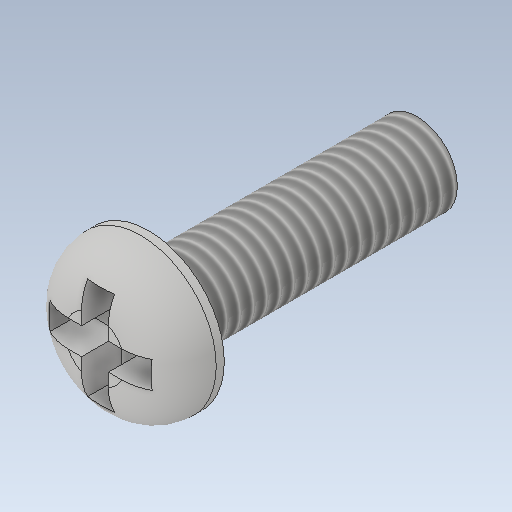
# Autodesk Inventor part: Винт М3х10
Saved by Autodesk Inventor 2020 (Build 240168000, 168)
## iProperties
Created: 2020-03-03
Part Number: Винт М3х10
Material: Типовые
Document SubType Name: Modeling
Designer: Leancher
Density: 1 g/cm^3
Appearance: По умолчанию
Author: Leancher
Autodesk Inventor part; units mm, degrees
ref_plane "YZ Plane" through (0, 0, 0) normal (1, 0, 0) x (0, 1, 0)
ref_plane "XZ Plane" through (0, 0, 0) normal (0, 1, 0) x (-1, 0, 0)
ref_plane "XY Plane" through (0, 0, 0) normal (0, 0, 1) x (1, 0, 0)
sketch "Эскиз1" plane through (0, 0, 0) normal (0, 0, 1) x (1, 0, 0)
  circle A0 centre (-4.8391, -17.7214) radius 1.5
  point P0 (0, 0)
  constraints: 1 centre point
extrude "Выдавливание1" add sketch "Эскиз1" against normal blind 10
sketch "Эскиз2" plane through (-4.8391, -17.7214, 0) normal (0, 0, 1) x (1, 0, 0)
  circle A0 centre (0, 0) radius 2.816
  point P0 (4.8391, 17.7214)
  constraints: 1 centre point
extrude "Выдавливание2" add sketch "Эскиз2" along normal blind 2
fillet "Сопряжение1" radius 1.7 1 edges at (-7.6551, -17.7214, 2)
sketch "Эскиз3" plane through (-4.8391, -17.7214, 2) normal (0, 0, 1) x (1, 0, 0)
  line L0 (-0.5, -1.9) -> (0.5, -1.9)
  line L1 (0.5, 1.9) -> (-0.5, 1.9)
  line L2 (1.9, -0.5) -> (1.9, 0.5)
  line L3 (-1.9, 0.5) -> (-1.9, -0.5)
  line L4 (-0.5, 1.9) -> (-0.5, 0.5)
  line L5 (-0.5, -0.5) -> (-0.5, -1.9)
  line L6 (1.9, 0.5) -> (0.5, 0.5)
  line L7 (-0.5, 0.5) -> (-1.9, 0.5)
  line L8 (0.5, -1.9) -> (0.5, -0.5)
  line L9 (0.5, 0.5) -> (0.5, 1.9)
  line L10 (-1.9, -0.5) -> (-0.5, -0.5)
  line L11 (0.5, -0.5) -> (1.9, -0.5)
  point P0 (4.8391, 17.7214)
  point P1 (0, 0)
  constraints: 24 end point, 10 parallel, 4 perpendicular, 3 horizontal
extrude "Выдавливание3" cut sketch "Эскиз3" against normal blind 1.5
thread "Резьба1" size "M3x0.5" class "6g" standard "ANSI Metric M Profile" full length
